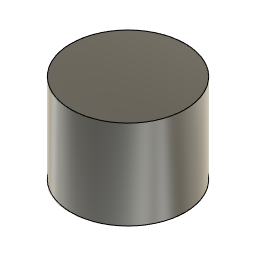
Gauge Placeholder v1 (Autodesk Fusion 360 design; units mm, degrees)
Autodesk Fusion 360 part; units mm, degrees
sketch "Sketch1" plane through (0, 0, 0) normal (0, 0, 1) x (1, 0, 0)
  circle A0 centre (0, 0) radius 32.0156
  constraint coincident A0.centre origin
extrude "Extrude1" add sketch "Sketch1" along normal blind 50
